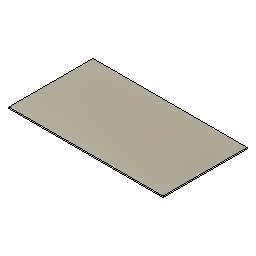
top half v8 (Autodesk Fusion 360 design; units mm, degrees)
Autodesk Fusion 360 part; units mm, degrees
sketch "Sketch1" plane through (0, 0, 0) normal (0, 0, 1) x (1, 0, 0)
  line L0 (115.5, -68.05) -> (-115.5, -68.05)
  line L1 (-115.5, -68.05) -> (-115.5, 68.05)
  line L2 (-115.5, 68.05) -> (115.5, 68.05)
  line L3 (115.5, 68.05) -> (115.5, -68.05)
  line L4 (115.5, -68.05) -> (-115.5, 68.05) construction
  line L5 (-115.5, -68.05) -> (115.5, 68.05) construction
  dimension "d1" = 136.1
  dimension "d2" = 231
  constraint horizontal L0
  constraint perpendicular L0 L1
  constraint parallel L0 L2
  constraint parallel L1 L3
  constraint coincident L4 origin
  constraint coincident L5 origin
  measures "d1" distance of L0.end L1.end
  measures "d2" distance of L0.start L0.end
extrude "Extrude1" add sketch "Sketch1" along normal blind 2
sketch "Sketch3" plane through (0, 0, 2) normal (0, 0, 1) x (-1, 0, 0)
  line L0 (-115.5, -68.05) -> (115.5, -68.05)
  line L1 (115.5, -68.05) -> (115.5, 68.05)
  line L2 (115.5, 68.05) -> (-115.5, 68.05)
  line L3 (-115.5, 68.05) -> (-115.5, -68.05)
move_face "OffsetFaces1" offset -5 1 faces at (38.5, -68.05, 0.6667)
extrude "Extrude2" cut 1 faces at (38.5, -63.05, 0.6667) along direction (0, 1, 0) blind 5
